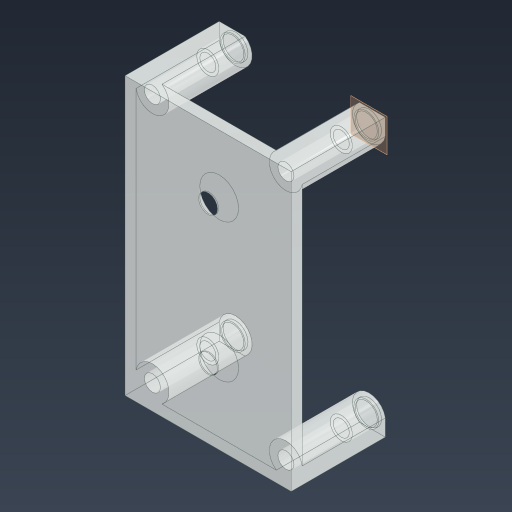
# Autodesk Inventor part: buck_holder
Saved by Autodesk Inventor 2023 (Build 270158000, 158)
## iProperties
Created: 2026-01-23
Part Number: buck_holder
Material: Glass
Document SubType Name: Modeling
Designer: szymo
Density: 2.18 g/cm^3
Appearance: Clear
Author: szymo
Autodesk Inventor part; units mm, degrees
ref_plane "YZ Plane" through (0, 0, 0) normal (1, 0, 0) x (0, 1, 0)
ref_plane "XZ Plane" through (0, 0, 0) normal (0, 1, 0) x (-1, 0, 0)
ref_plane "XY Plane" through (0, 0, 0) normal (0, 0, 1) x (1, 0, 0)
ref_plane "Work Plane1" through (0, 0, -14.5) normal (0, 0, 1) x (1, 0, 0)
sketch "Sketch1" plane through (0, 0, -14.5) normal (0, 0, 1) x (1, 0, 0)
  arc A0 (10.3187, 25) -> (15, 22.0046) centre (12.05, 22.55) ccw projected
  line L0 (15, 22.0046) -> (15, 25) projected
  line L1 (15, 25) -> (10.3187, 25) projected
  circle A1 centre (12.05, 22.55) radius 1.45 projected
  arc A2 (15, -22.0046) -> (10.3187, -25) centre (12.05, -22.55) ccw projected
  line L2 (10.3187, -25) -> (15, -25) projected
  line L3 (15, -25) -> (15, -22.0046) projected
  circle A3 centre (12.05, -22.55) radius 1.45 projected
  arc A4 (-10.3187, -25) -> (-15, -22.0046) centre (-12.05, -22.55) ccw projected
  line L4 (-15, -22.0046) -> (-15, -25) projected
  line L5 (-15, -25) -> (-10.3187, -25) projected
  circle A5 centre (-12.05, -22.55) radius 1.45 projected
  circle A6 centre (-12.05, 22.55) radius 1.45 projected
  arc A7 (-15, 22.0046) -> (-10.3187, 25) centre (-12.05, 22.55) ccw projected
  line L6 (-10.3187, 25) -> (-15, 25) projected
  line L7 (-15, 25) -> (-15, 22.0046) projected
  point P0 (0, 0)
extrude "Extrusion1" add sketch "Sketch1" along normal blind 15
sketch "Sketch2" plane through (0, 0, 0.5) normal (0, 0, 1) x (1, 0, 0)
  line L0 (15, 22.0046) -> (15, 25) projected
  line L1 (15, 25) -> (10.3187, 25) projected
  arc A0 (10.3187, 25) -> (15, 22.0046) centre (12.05, 22.55) ccw projected
  circle A1 centre (12.05, 22.55) radius 1.45 projected
  line L2 (10.3187, -25) -> (15, -25) projected
  line L3 (15, -25) -> (15, -22.0046) projected
  arc A2 (15, -22.0046) -> (10.3187, -25) centre (12.05, -22.55) ccw projected
  circle A3 centre (12.05, -22.55) radius 1.45 projected
  line L4 (-15, -22.0046) -> (-15, -25) projected
  line L5 (-15, -25) -> (-10.3187, -25) projected
  arc A4 (-10.3187, -25) -> (-15, -22.0046) centre (-12.05, -22.55) ccw projected
  circle A5 centre (-12.05, -22.55) radius 1.45 projected
  line L6 (-10.3187, 25) -> (-15, 25) projected
  line L7 (-15, 25) -> (-15, 22.0046) projected
  arc A6 (-15, 22.0046) -> (-10.3187, 25) centre (-12.05, 22.55) ccw projected
  circle A7 centre (-12.05, 22.55) radius 1.45 projected
  line L8 (15, 25) -> (10.3187, 25) projected
  line L9 (-15, -25) -> (-10.3187, -25) projected
  line L10 (15, 25) -> (-15, 25)
  line L11 (-15, 25) -> (-15, -25)
  line L12 (-15, -25) -> (15, -25)
  line L13 (15, -25) -> (15, 25)
  point P0 (0, 0)
  constraints: 8 end point, 2 parallel, 1 horizontal, 1 perpendicular
extrude "Extrusion2" add sketch "Sketch2" along normal blind 2 contours A0 L1 L0 | L13 A2 L12 A4 L11 A6 L10 A0 | L3 L2 A2 | A6 L7 L6 | L5 L4 A4 | A1 | A3 | A5 | A7
sketch "Sketch3" plane through (0, 0, -14.5) normal (0, 0, -1) x (-1, 0, 0)
  circle A0 centre (12.05, 22.55) radius 1.45 projected
  circle A1 centre (-12.05, 22.55) radius 1.45 projected
  circle A2 centre (-12.05, -22.55) radius 1.45 projected
  circle A3 centre (12.05, -22.55) radius 1.45 projected
  line L0 (15, -25) -> (-15, -25) projected
  line L1 (15, 25) -> (15, -25) projected
  line L2 (-15, 25) -> (15, 25) projected
  line L3 (-15, -25) -> (-15, 25) projected
  circle A4 centre (12.05, -22.55) radius 1.45 projected
  circle A5 centre (-12.05, -22.55) radius 1.45 projected
  circle A6 centre (-12.05, 22.55) radius 1.45 projected
  circle A7 centre (12.05, 22.55) radius 1.45 projected
  point P0 (0, 0)
  constraints: 4 coincident
hole "Hole1" at (-12.05, -22.55, -14.5) at (12.05, -22.55, -14.5) at (12.05, 22.55, -14.5) at (-12.05, 22.55, -14.5) direction (0, 0, 1) diameter 4 depth 5 counterbore diameter 4.5 counterbore depth 0.5
sketch "Sketch4" plane through (0, 0, 0.5) normal (0, 0, -1) x (-1, 0, 0)
  circle A0 centre (12.05, 22.55) radius 1.45 projected
  circle A1 centre (-12.05, 22.55) radius 1.45 projected
  circle A2 centre (-12.05, -22.55) radius 1.45 projected
  circle A3 centre (12.05, -22.55) radius 1.45 projected
  line L0 (15, -25) -> (-15, -25) projected
  line L1 (15, 25) -> (15, -25) projected
  line L2 (-15, 25) -> (15, 25) projected
  line L3 (-15, -25) -> (-15, 25) projected
  line L4 (0, 12.5) -> (0, -12.5)
  point P0 (0, 0)
  dimension "d11" = 12.5
  dimension "d12" = 12.5
  dimension "d13" = 12.5
  dimension "d14" = 12.5
  constraints: 2 end point, 1 midpoint, 1 vertical
  measures "d11" distance from line of L2 L4.start
  measures "d12" distance of point (0, 0) L4.start
  measures "d13" distance of L4.end point (0, 0)
  measures "d14" distance from line of L0 L4.end
hole "Hole2" at (0, 12.5, 0.5) at (0, -12.5, 0.5) direction (0, 0, 1) diameter 3.4 depth 5 countersink diameter 7 countersink angle 90 clearance for "Countersunk Flat Head Screw ISO 2009/7046" size "M3" standard "ISO"
equation "\"d11\" = d12"
equation "\"d13\" = d14"
body "Solid1"
